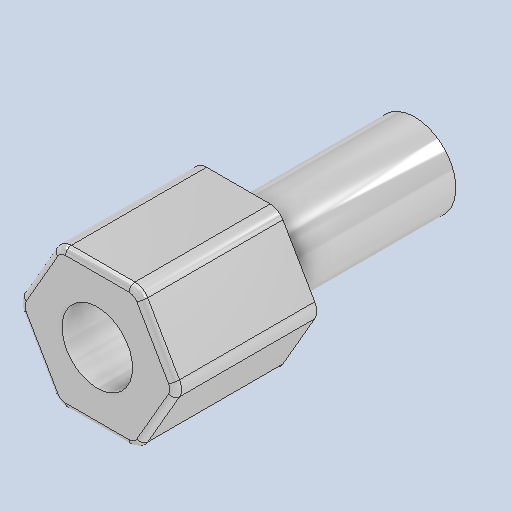
# Autodesk Inventor part: 5207953-3
Saved by Autodesk Inventor 2024.2 (Build 282272000, 272)
## iProperties
Created: 2020-07-14
Part Number: 5207953-3
Material: Generic
Document SubType Name: Modeling
Designer: CASE-SMALL2
Density: 1 g/cm^3
Appearance: Default
Author: CASE-SMALL2
Autodesk Inventor part; units mm, degrees
ref_plane "YZ Plane" through (0, 0, 0) normal (1, 0, 0) x (0, 1, 0)
ref_plane "XZ Plane" through (0, 0, 0) normal (0, 1, 0) x (-1, 0, 0)
ref_plane "XY Plane" through (0, 0, 0) normal (0, 0, 1) x (1, 0, 0)
sketch "Sketch1" plane through (0, 0, 0) normal (0, 0, 1) x (1, 0, 0)
  line L0 (2.7424, 0) -> (1.3712, -2.375)
  line L1 (1.3712, -2.375) -> (-1.3712, -2.375)
  line L2 (-1.3712, -2.375) -> (-2.7424, 0)
  line L3 (-2.7424, 0) -> (-1.3712, 2.375)
  line L4 (-1.3712, 2.375) -> (1.3712, 2.375)
  line L5 (1.3712, 2.375) -> (2.7424, 0)
  point P0 (0, 0)
  point P1 (0, 0)
  dimension "d0" = 4.75
  constraints: 12 end point, 1 coincident, 13 other
  measures "d0" distance between parallel lines of L1 L4
extrude "Extrusion1" add sketch "Sketch1" along normal blind 4.8
sketch "Sketch2" plane through (0, 0, 0) normal (0, 0, -1) x (-1, 0, 0)
  circle A0 centre (0, 0) radius 1.4
  dimension "d3" = 2.8
  constraints: 1 centre point, 1 coincident
  measures "d3" diameter of A0
extrude "Extrusion2" add sketch "Sketch2" along normal blind 6
sketch "Sketch3" plane through (0, 0, 4.8) normal (0, 0, 1) x (1, 0, 0)
  circle A0 centre (0, 0) radius 1.2
  dimension "d6" = 2.4
  constraints: 1 centre point, 1 coincident
  measures "d6" diameter of A0
extrude "Extrusion3" cut sketch "Sketch3" against normal blind 4
fillet "Fillet1" radius 0.5 6 edges at (-2.7424, 0, 2.4) (-1.3712, -2.375, 2.4) (1.3712, -2.375, 2.4) (2.7424, 0, 2.4) (1.3712, 2.375, 2.4) (-1.3712, 2.375, 2.4)
fillet "Fillet2" radius 0.2 12 edges at (-2.0568, 1.1875, 4.8) (-2.6651, 0, 4.8) (-2.0568, -1.1875, 4.8) (-1.3325, -2.308, 4.8) (0, -2.375, 4.8) (1.3325, -2.308, 4.8) (2.0568, -1.1875, 4.8) (2.6651, 0, 4.8) (2.0568, 1.1875, 4.8) (1.3325, 2.308, 4.8) (0, 2.375, 4.8) (-1.3325, 2.308, 4.8)
body "Solid1"
